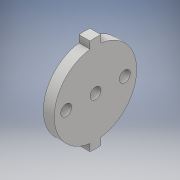
# Autodesk Inventor part: tapa
Saved by Autodesk Inventor 2018 (Build 220112000, 112)
## iProperties
Created: 2020-03-11
Part Number: tapa
Material: Genérico
Document SubType Name: Modeling
Designer: sala.ceri
Density: 1 g/cm^3
Appearance: Valor por defecto
Author: sala.ceri
Autodesk Inventor part; units mm, degrees
ref_plane "YZ Plane" through (0, 0, 0) normal (1, 0, 0) x (0, 1, 0)
ref_plane "XZ Plane" through (0, 0, 0) normal (0, 1, 0) x (-1, 0, 0)
ref_plane "XY Plane" through (0, 0, 0) normal (0, 0, 1) x (1, 0, 0)
sketch "Boceto1" plane through (0, 0, 0) normal (1, 0, 0) x (0, 1, 0)
  line L0 (1.5, -11.1496) -> (1.5, -13.0893)
  line L1 (-1.5, -11.1496) -> (-1.5, -13.0893)
  line L2 (-1.5, 11.1496) -> (-1.5, 13.0893)
  line L3 (1.5, 11.1496) -> (1.5, 13.0893)
  arc A0 (1.5, 13.0893) -> (-1.5, 13.0893) centre (0, 0) ccw
  arc A1 (-1.5, -13.0893) -> (1.5, -13.0893) centre (0, 0) ccw
  arc A2 (-1.5, 11.1496) -> (-1.5, -11.1496) centre (0, 0) ccw
  arc A3 (1.5, -11.1496) -> (1.5, 11.1496) centre (0, 0) ccw
  constraints: 8 end point, 8 point on circle, 4 centre point, 1 coincident, 1 parallel, 1 vertical
extrude "Extrusión1" add sketch "Boceto1" along normal blind 3
sketch "Boceto2" plane through (3, 0, 0) normal (1, 0, 0) x (0, 0, -1)
  circle A0 centre (0, 8) radius 1.5
  circle A1 centre (0, -8) radius 1.5
  dimension "d14" = 3
  dimension "d15" = 3
  constraints: 2 centre point
  measures "d14" diameter of A0
  measures "d15" diameter of A1
extrude "Extrusión2" cut sketch "Boceto2" against normal blind 3
sketch "Boceto3" plane through (3, 0, 0) normal (1, 0, 0) x (0, 0, -1)
  circle A0 centre (0, 0) radius 1.5
  dimension "d18" = 3
  constraints: 1 centre point, 1 coincident
  measures "d18" diameter of A0
extrude "Extrusión3" cut sketch "Boceto3" against normal blind 10
